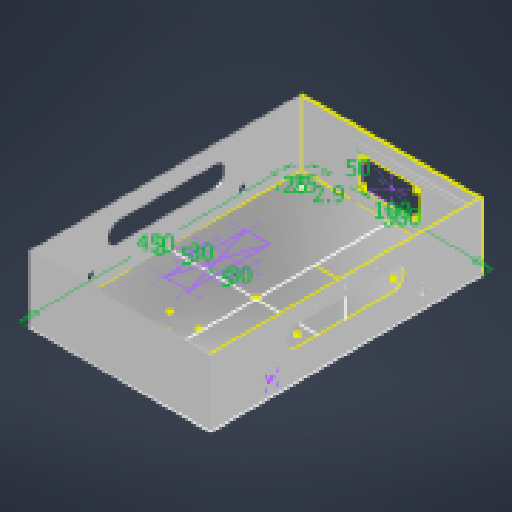
# Autodesk Inventor part: AMR_Base_Box_V2
Saved by Autodesk Inventor 2026.2 (Build 302298010, 298A)
## iProperties
Created: 2026-03-25
Part Number: AMR_Base_Box_V2
Material: Aluminum 6061
Document SubType Name: Modeling
Designer: Srishanth Dhondy
Density: 2.7 g/cm^3
Appearance: Aluminum - Flat
Mass: 2297.89 g
Surface Area: 5654.69 cm^2
Volume: 851.072 cm^3
Author: Srishanth Dhondy
Autodesk Inventor part; units mm, degrees
ref_plane "YZ Plane" through (0, 0, 0) normal (1, 0, 0) x (0, 1, 0)
ref_plane "XZ Plane" through (0, 0, 0) normal (0, 1, 0) x (-1, 0, 0)
ref_plane "XY Plane" through (0, 0, 0) normal (0, 0, 1) x (1, 0, 0)
sketch "Sketch1" plane through (0, 0, 0) normal (0, 1, 0) x (-1, 0, 0)
  line L0 (-150, 225) -> (150, 225)
  line L1 (150, 225) -> (150, -225)
  line L2 (150, -225) -> (-150, -225)
  line L3 (-150, -225) -> (-150, 225)
  line L4 (-150, 225) -> (150, -225) construction
  line L5 (150, 225) -> (-150, -225) construction
  line L6 (147, -222) -> (147, 222)
  line L7 (147, 222) -> (-147, 222)
  line L8 (-147, 222) -> (-147, -222)
  line L9 (-147, -222) -> (147, -222)
  point P0 (0, 0)
  dimension "Base_Width" = 300
  dimension "Base_Length" = 450
  dimension "Base_Wall_Thickness" = 3
  constraints: 20 end point, 4 parallel, 2 midpoint, 2 perpendicular, 1 horizontal, 3 other
  measures "Base_Width" distance of L1.end L2.end
  measures "Base_Length" distance of L0.end L1.end
  measures "Base_Wall_Thickness" distance between parallel lines of L1 L6
extrude "Extrusion1" add sketch "Sketch1" along normal blind 3 contours L0 L1 L2 L3 | L9 L8 L7 L6
extrude "Extrusion2" add sketch "Sketch1" along normal blind 110
sketch "Sketch2" plane through (150, 0, 225) normal (1, 0, 0) x (0, 0, -1)
  line L0 (0, 0) -> (450, 0) projected
  line L1 (450, 0) -> (450, 110) projected
  line L2 (0, 110) -> (450, 110) projected
  line L3 (0, 0) -> (0, 110) projected
  line L4 (0, 25) -> (450, 25)
  line L5 (100, 25) -> (114, 25) construction
  line L6 (225, 110) -> (225, 0) construction
  circle A0 centre (100, 25) radius 19.5
  circle A1 centre (100, 25) radius 6
  circle A2 centre (100, 25) radius 7.75
  circle A3 centre (84.5, 25) radius 1.75
  circle A4 centre (100, 40.5) radius 1.75
  circle A5 centre (100, 9.5) radius 1.75
  circle A6 centre (115.5, 25) radius 1.75
  line L7 (350, 25) -> (336, 25) construction
  circle A7 centre (350, 25) radius 19.5
  circle A8 centre (350, 25) radius 6
  circle A9 centre (350, 25) radius 7.75
  circle A10 centre (365.5, 25) radius 1.75
  circle A11 centre (350, 40.5) radius 1.75
  circle A12 centre (350, 9.5) radius 1.75
  circle A13 centre (334.5, 25) radius 1.75
  point P0 (119.5, 25)
  point P1 (80.5, 25)
  point P2 (100, 5.5)
  point P3 (100, 44.5)
  point P4 (330.5, 25)
  point P5 (369.5, 25)
  point P6 (350, 5.5)
  point P7 (350, 44.5)
  dimension "d138" = 39
  dimension "d139" = 12
  dimension "d140" = 15.5
  dimension "d141" = 3.5
  dimension "d143" = 3.5
  dimension "d144" = 3.5
  dimension "d145" = 3.5
  constraints: 22 coincident, 22 symmetric about line, 14 centre point, 8 end point, 8 point on circle, 7 point on line, 2 perpendicular, 1 horizontal, 1 midpoint, 7 other
  measures "d138" diameter of A0
  measures "d139" diameter of A1
  measures "d140" diameter of A2
  measures "d141" diameter of A3
  measures "d143" diameter of A4
  measures "d144" diameter of A5
  measures "d145" diameter of A6
sketch "Sketch3" plane through (0, 3, 0) normal (0, 1, 0) x (1, 0, 0)
  line L0 (-147, 222) -> (-147, -222) projected
  line L1 (-147, -222) -> (147, -222) projected
  line L2 (147, -222) -> (147, 222) projected
  line L3 (147, 222) -> (-147, 222) projected
  point P0 (0, 0)
sketch "Sketch7" plane through (150, 0, 225) normal (1, 0, 0) x (0, 0, -1)
  line L0 (145, 65.000074) -> (305, 65.000074) construction
  line L1 (145, 47.500074) -> (305, 47.500074)
  line L2 (305, 82.500074) -> (145, 82.500074)
  arc A0 (145, 82.500074) -> (145, 47.500074) centre (145, 65.000074) ccw
  arc A1 (305, 47.500074) -> (305, 82.500074) centre (305, 65.000074) ccw
  point P0 (225, 0)
  point P1 (225, 65.000074)
  dimension "Handle_Slot_Length" = 80
  dimension "Handle_Cutout_Height" = 35
  constraints: 8 end point, 4 point on circle, 4 tangent, 2 centre point, 1 horizontal, 1 midpoint, 1 parallel
  measures "Handle_Slot_Length" distance of point (225, 65) L0.end
  measures "Handle_Cutout_Height" diameter of A1
extrude "Extrusion3" cut sketch "Sketch7" against normal through all
sketch "Sketch9" plane through (150, 0, -225) normal (0, 0, -1) x (-1, 0, 0)
  line L0 (0, 0) -> (300, 0) projected
  line L1 (300, 0) -> (300, 110) projected
  line L2 (0, 110) -> (300, 110) projected
  line L3 (0, 0) -> (0, 110) projected
  line L4 (100, 75) -> (200, 75)
  line L5 (200, 75) -> (200, 25)
  line L6 (200, 25) -> (100, 25)
  line L7 (100, 25) -> (100, 75)
  line L8 (100, 75) -> (200, 25) construction
  line L9 (200, 75) -> (100, 25) construction
  point P0 (150, 0)
  point P1 (150, 50)
  point P2 (150, 50)
  dimension "Rear_Port_Width" = 100
  dimension "Rear_Port_Height" = 50
  constraints: 12 end point, 2 midpoint, 2 parallel, 1 coincident, 1 horizontal, 1 perpendicular
  measures "Rear_Port_Width" distance of L5.end L6.end
  measures "Rear_Port_Height" distance of L4.end L5.end
sketch "Sketch10" plane through (150, 0, -225) normal (0, 0, -1) x (-1, 0, 0)
  line L0 (100.000061, 70.00003) -> (100.000061, 30.000011)
  line L1 (105.000061, 25.000011) -> (195.003813, 25.000011)
  line L2 (200.003813, 30.000011) -> (200.003813, 70.00003)
  line L3 (195.003813, 75.00003) -> (105.000061, 75.00003)
  arc A0 (105.000061, 75.00003) -> (100.000061, 70.00003) centre (105.000061, 70.00003) ccw
  arc A1 (100.000061, 30.000011) -> (105.000061, 25.000011) centre (105.000061, 30.000011) ccw
  arc A2 (195.003813, 25.000011) -> (200.003813, 30.000011) centre (195.003813, 30.000011) ccw
  arc A3 (200.003813, 70.00003) -> (195.003813, 75.00003) centre (195.003813, 70.00003) ccw
  point P0 (150, 0)
  point P1 (200.003813, 75.00003)
  point P2 (100.003813, 75.00003)
  dimension "d48" = 100
  dimension "Rear_Port_Fillet" = 5
  constraints: 8 end point, 8 point on circle, 8 tangent, 4 centre point, 3 equal radius, 3 perpendicular, 3 point on line, 1 vertical
  measures "d48" distance of point (200.004, 75) point (100.004, 75)
  measures "Rear_Port_Fillet" radius of A0
extrude "Extrusion4" cut sketch "Sketch10" against normal blind 3
sketch "Sketch11" plane through (147, 3, 222) normal (-1, 0, 0) x (0, 0, 1)
  line L0 (-302, 79.500074) -> (-142, 79.500074)
  arc A0 (-142, 44.500074) -> (-142, 79.500074) centre (-142, 62.000074) ccw
  line L1 (-142, 44.500074) -> (-302, 44.500074)
  arc A1 (-302, 79.500074) -> (-302, 44.500074) centre (-302, 62.000074) ccw
  circle A2 centre (-106.899495, 31.899495) radius 1.75
  circle A3 centre (-87.100505, 12.100505) radius 1.75
  circle A4 centre (-106.899495, 12.100505) radius 1.75
  circle A5 centre (-87.100505, 31.899495) radius 1.75
  circle A6 centre (-97, 22) radius 6
  line L2 (0, 0) -> (-444, 0)
  line L3 (0, 0) -> (0, 107)
  line L4 (-444, 107) -> (0, 107)
  line L5 (-444, 0) -> (-444, 107)
  line L6 (0, 107) -> (-444, 107)
  line L7 (-222, 107) -> (-222, -3)
  line L8 (-222, -3) -> (-222, 107)
  constraints: 4 end point, 2 perpendicular, 1 midpoint
sketch "Sketch13" plane through (-147, 3, -222) normal (0, 0, 1) x (1, 0, 0)
  line L0 (191.999939, 22.000011) -> (101.996187, 22.000011)
  arc A0 (96.996187, 27.000011) -> (101.996187, 22.000011) centre (101.996187, 27.000011) ccw
  line L1 (96.996187, 27.000011) -> (96.996187, 67.00003)
  arc A1 (101.996187, 72.00003) -> (96.996187, 67.00003) centre (101.996187, 67.00003) ccw
  line L2 (101.996187, 72.00003) -> (191.999939, 72.00003)
  arc A2 (196.999939, 67.00003) -> (191.999939, 72.00003) centre (191.999939, 67.00003) ccw
  line L3 (196.999939, 67.00003) -> (196.999939, 27.000011)
  arc A3 (191.999939, 22.000011) -> (196.999939, 27.000011) centre (191.999939, 27.000011) ccw
  line L4 (294, 0) -> (0, 0)
  line L5 (294, 0) -> (294, 107)
  line L6 (0, 107) -> (294, 107)
  line L7 (0, 0) -> (0, 107)
  point P0 (147, -3)
sketch "Sketch14" plane through (-147, 3, -222) normal (0, 0, 1) x (1, 0, 0)
  line L0 (294, 0) -> (0, 0)
  line L1 (294, 0) -> (294, 107)
  line L2 (0, 0) -> (0, 107)
  line L3 (297, 107) -> (-3, 107)
  line L4 (147, 107) -> (147, 0)
  line L5 (101.996187, 13.5) -> (293.998542, 13.5)
  line L6 (293.998542, 13.5) -> (293.998542, 3.5)
  line L7 (293.998542, 3.5) -> (101.996187, 3.5)
  line L8 (101.996187, 3.5) -> (101.996187, 13.5)
  line L9 (0, 53.5) -> (294, 53.5)
  line L10 (101.996187, 90.5) -> (293.996187, 90.5)
  line L11 (293.996187, 90.5) -> (293.996187, 80.5)
  line L12 (293.996187, 80.5) -> (101.996187, 80.5)
  line L13 (101.996187, 80.5) -> (101.996187, 90.5)
  point P0 (101.996187, 22.000011)
  point P1 (147, -3)
  point P2 (101.996187, 22.000011)
  point P3 (0.001458, 3.5)
  point P4 (0.001458, 3.5)
  point P5 (192.003813, 13.5)
  point P6 (0.003813, 80.5)
  point P7 (0.003813, 80.5)
  point P8 (192.003813, 90.5)
  dimension "d52" = 192
  dimension "d53" = 10
  constraints: 20 end point, 5 coincident, 4 midpoint, 4 parallel, 4 symmetric about line, 2 horizontal, 2 perpendicular, 1 point on line
  measures "d52" distance of L11.end L12.end
  measures "d53" distance of L12.end L10.start
sketch "Sketch14 outline for Extrusion5" plane through (-147, 3, -222) normal (0, 0, 1) x (1, 0, 0)
  line L0 (293.998542, 3.5) -> (293.998542, 13.5)
  line L1 (101.996187, 3.5) -> (293.998542, 3.5)
  line L2 (101.996187, 13.5) -> (101.996187, 3.5)
  line L3 (293.998542, 13.5) -> (101.996187, 13.5)
  line L4 (293.996187, 80.5) -> (293.996187, 90.5)
  line L5 (101.996187, 80.5) -> (293.996187, 80.5)
  line L6 (101.996187, 90.5) -> (101.996187, 80.5)
  line L7 (293.996187, 90.5) -> (101.996187, 90.5)
extrude "Extrusion5" add sketch "Sketch14 outline for Extrusion5" along normal blind 3.5
sketch "Sketch15" plane through (-147, 3, -218.5) normal (0, 0, 1) x (1, 0, 0)
  line L0 (101.996187, 90.5) -> (101.996187, 80.5)
  line L1 (101.996187, 80.5) -> (293.996187, 80.5)
  line L2 (293.996187, 80.5) -> (293.996187, 90.5)
  line L3 (101.996187, 85.5) -> (293.996187, 85.5)
  line L4 (293.996187, 85.5) -> (293.996187, 80.5)
  line L5 (293.996187, 80.5) -> (101.996187, 80.5)
  line L6 (101.996187, 80.5) -> (101.996187, 85.5)
  line L7 (293.998542, 13.5) -> (101.996187, 13.5)
  line L8 (293.998542, 3.5) -> (293.998542, 13.5)
  line L9 (101.996187, 13.5) -> (293.998542, 13.5)
  line L10 (293.998542, 13.5) -> (293.998542, 8.5)
  line L11 (293.998542, 8.5) -> (101.996187, 8.5)
  line L12 (101.996187, 8.5) -> (101.996187, 13.5)
  point P0 (147, -3)
  constraints: 16 end point, 4 parallel, 2 horizontal, 2 midpoint, 2 perpendicular
extrude "Extrusion6" add sketch "Sketch15" along normal blind 2
sketch "Sketch17" plane through (0, 3, 0) normal (0, 1, 0) x (1, 0, 0)
  line L0 (-147, 222) -> (-147, -222) projected
  line L1 (-147, -222) -> (147, -222) projected
  line L2 (147, -222) -> (147, 222) projected
  line L3 (147, 222) -> (-147, 222) projected
  circle A0 centre (-120.55, 195.55) radius 1.45
  line L4 (-147, 0) -> (147, 0)
  line L5 (0, -222) -> (0, 222)
  circle A1 centre (-120.55, -195.55) radius 1.45
  line L6 (0, 222) -> (0, -222)
  circle A2 centre (-120.55, -195.55) radius 1.45
  circle A3 centre (120.55, 195.55) radius 1.45
  circle A4 centre (120.55, -195.55) radius 1.45
  line L7 (0, 222) -> (0, -222)
  point P0 (0, 0)
  dimension "d58" = 2.9
  dimension "d59" = 25
  dimension "d60" = 25
  constraints: 8 end point, 6 symmetric about line, 5 centre point, 4 midpoint, 1 perpendicular, 4 other
  measures "d58" diameter of A0
  measures "d59" distance edge to line of A0 L3
  measures "d60" distance edge to line of A0 L0
extrude "Extrusion7" cut sketch "Sketch17" against normal blind 110 contours A0
extrude "Extrusion8" cut sketch "Sketch17" against normal blind 110 contours A1
extrude "Extrusion9" cut sketch "Sketch17" against normal blind 110 contours A4
extrude "Extrusion10" cut sketch "Sketch17" against normal blind 110 contours A3
sketch "Sketch18" plane through (-147, 3, -222) normal (1, 0, 0) x (0, 0, -1)
  line L0 (-142, 79.500074) -> (-285.5, 79.500074)
  line L1 (-285.5, 79.500074) -> (-285.5, 101.1)
  line L2 (-158.5, 79.503299) -> (-285.5, 79.503299)
  line L3 (-285.5, 79.503299) -> (-285.5, 102.503299)
  line L4 (-285.5, 102.503299) -> (-158.5, 102.503299)
  line L5 (-158.5, 102.503299) -> (-158.5, 79.503299)
  line L6 (-158.5, 79.503299) -> (-285.5, 102.503299) construction
  line L7 (-285.5, 79.503299) -> (-158.5, 102.503299) construction
  circle A0 centre (-272.8, 92.853299) radius 2.25
  circle A1 centre (-171.2, 92.978299) radius 2.25
  point P0 (-222, -3)
  point P1 (-302, 101.1)
  point P2 (-302, 101.1)
  point P3 (-302, 101.1)
  point P4 (-302, 101.1)
  point P5 (-142, 101.1)
  point P6 (-142, 101.1)
  point P7 (-142, 101.1)
  point P8 (-158.5, 101.1)
  point P9 (-222, 93.25)
  point P10 (-222, 91.003299)
  dimension "d70" = 127
  dimension "d71" = 23
  dimension "d73" = 4.5
  dimension "d74" = 11.1
  dimension "d75" = 12.7
  dimension "d76" = 4.5
  dimension "d77" = 13.475
  dimension "d78" = 12.7
  constraints: 16 end point, 5 coincident, 2 centre point, 2 midpoint, 2 parallel, 1 horizontal, 1 perpendicular
  measures "d70" distance of L3.end L4.end
  measures "d71" distance of L2.end L3.end
  measures "d73" diameter of A0
  measures "d74" distance edge to line of A0 L2
  measures "d75" distance from line of L3 A0.centre
  measures "d76" diameter of A1
  measures "d77" distance from line of L2 A1.centre
  measures "d78" distance from line of L5 A1.centre
extrude "Extrusion11" cut sketch "Sketch18" along normal through all both and the other way through all contours A0 | A1
sketch "Sketch19" plane through (-147, 3, -222) normal (1, 0, 0) x (0, 0, -1)
  circle A0 centre (-222, 92.978299) radius 2.25
  point P0 (-222, -3)
  dimension "d81" = 4.5
  constraints: 1 centre point, 1 coincident
  measures "d81" diameter of A0
extrude "Extrusion12" cut sketch "Sketch19" along normal through all both and the other way through all
sketch "Sketch22" plane through (147, 3, 222) normal (-1, 0, 0) x (0, 0, 1)
  line L0 (-444, 0) -> (-444, 107) projected
  line L1 (-444, 80.5) -> (-440.5, 80.5)
  line L2 (-440.5, 80.5) -> (-440.5, 13.5)
  line L3 (-440.5, 13.5) -> (-444, 13.5)
  line L4 (-444, 13.5) -> (-444, 80.5)
  point P0 (-222, -3)
  dimension "d84" = 3.5
  constraints: 8 end point, 2 parallel, 1 horizontal, 1 perpendicular
  measures "d84" distance of L2.end L3.end
extrude "Extrusion13" add sketch "Sketch22" along normal blind 10
sketch "Sketch23" plane through (-147, 110, -222) normal (0, 0, 1) x (1, 0, 0)
  line L0 (101.996187, -26.5) -> (101.996187, -16.5)
  line L1 (101.996187, -26.5) -> (293.996187, -26.5)
  line L2 (101.996187, -26.5) -> (95.696187, -26.5)
  line L3 (95.696187, -26.5) -> (95.696187, -16.5)
  line L4 (95.696187, -16.5) -> (101.996187, -16.5)
  line L5 (101.996187, -16.5) -> (101.996187, -26.5)
  line L6 (101.996187, -21.5) -> (293.996187, -21.5)
  line L7 (101.996187, -21.5) -> (105.795872, -23.663742)
  line L8 (101.996187, -21.5) -> (95.696187, -21.5)
  line L9 (95.696187, -21.5) -> (101.996187, -21.5)
  point P0 (147, -110)
  dimension "d87" = 6.3
  dimension "d88" = 10
  dimension "d89" = 6.3
  constraints: 14 end point, 2 parallel, 1 horizontal, 1 midpoint, 1 perpendicular
  measures "d87" distance of L3.end L4.end
  measures "d88" distance of L2.end L3.end
  measures "d89" distance of L6.start L8.end
extrude "Extrusion14" add sketch "Sketch23" along normal blind 5.5 contours L2 L3 L8 L0
extrude "Extrusion15" add sketch "Sketch23" along normal blind 3.5
sketch "Sketch24" plane through (-147, 110, -222) normal (0, 0, 1) x (1, 0, 0)
  line L0 (101.996187, -103.5) -> (101.996187, -93.5)
  line L1 (101.996187, -103.5) -> (95.696187, -103.5)
  line L2 (95.696187, -103.5) -> (95.696187, -93.5)
  line L3 (95.696187, -93.5) -> (101.996187, -93.5)
  line L4 (101.996187, -93.5) -> (101.996187, -103.5)
  line L5 (101.996187, -98.5) -> (105.945782, -102.881271)
  line L6 (101.996187, -98.5) -> (95.696, -98.5)
  point P0 (147, -110)
  point P1 (95.696187, -98.5)
  dimension "d94" = 6.3
  constraints: 12 end point, 2 parallel, 2 perpendicular, 1 horizontal, 1 midpoint
  measures "d94" distance of L2.end L3.end
extrude "Extrusion16" add sketch "Sketch24" along normal blind 5.5 contours L6 L2 L3 L0
extrude "Extrusion17" add sketch "Sketch24" along normal blind 3.5 contours L1 L2 L6 L0
sketch "Sketch25" plane through (-147, 110, -222) normal (0, 0, 1) x (1, 0, 0)
  line L0 (95.696187, -103.5) -> (95.696187, -93.5)
  line L1 (95.696187, -93.5) -> (284, -93.5)
  line L2 (284, -26.5) -> (95.696187, -26.5)
  line L3 (95.696187, -26.5) -> (95.696187, -16.5)
  line L4 (95.696187, -16.5) -> (293.996187, -16.5)
  line L5 (293.998542, -103.5) -> (95.696187, -103.5)
  line L6 (95.696187, -103.5) -> (85.696, -103.5)
  line L7 (85.696, -103.5) -> (85.696, -16.5)
  line L8 (85.696, -16.5) -> (95.696187, -16.5)
  line L9 (95.696187, -16.5) -> (95.696187, -103.5)
  point P0 (147, -110)
  point P1 (85.696, -26.5)
  point P2 (85.696, -93.5)
  point P3 (85.696, -100.25)
  constraints: 8 end point, 4 point on line, 2 parallel, 1 horizontal, 1 perpendicular
extrude "Extrusion18" add sketch "Sketch25" along normal blind 5.5
sketch "Sketch26" plane through (0, 3, 0) normal (0, 1, 0) x (1, 0, 0)
  line L0 (-1.867084, -74) -> (-51.867084, -74)
  line L1 (-54.867084, -77) -> (-54.867084, -150)
  line L2 (-51.867084, -153) -> (-1.867084, -153)
  line L3 (1.132916, -150) -> (1.132916, -77)
  arc A0 (-54.867084, -150) -> (-51.867084, -153) centre (-51.867084, -150) ccw
  arc A1 (-1.867084, -153) -> (1.132916, -150) centre (-1.867084, -150) ccw
  arc A2 (1.132916, -77) -> (-1.867084, -74) centre (-1.867084, -77) ccw
  arc A3 (-51.867084, -74) -> (-54.867084, -77) centre (-51.867084, -77) ccw
  line L4 (-26.867084, -74) -> (-26.867084, -153)
  line L5 (-54.867084, -113.5) -> (1.132916, -113.5)
  circle A4 centre (-51.367, -149.5) radius 1.35
  circle A5 centre (-2.367168, -149.5) radius 1.35
  circle A6 centre (-51.367, -77.5) radius 1.35 construction
  circle A7 centre (-2.367168, -77.5) radius 1.35
  circle A8 centre (-2.367168, -77.5) radius 1.35
  circle A9 centre (-51.367, -149.5) radius 1.35
  circle A10 centre (-2.367168, -149.5) radius 1.35
  circle A11 centre (-51.367, -77.5) radius 1.35
  line L6 (-51.367, -77.5) -> (-51.367, -149.5)
  circle A12 centre (-51.367, -91.5) radius 1.35
  circle A13 centre (-2.367168, -91.5) radius 1.35
  point P0 (0, 0)
  point P1 (-64, -151.953345)
  point P2 (-14, -151.953345)
  point P3 (-54.867084, -153)
  point P4 (-54.867084, -74)
  point P5 (-60.5, -150)
  point P6 (-61, -149.5)
  point P7 (-51.367, -150)
  point P8 (-51.867084, -149.5)
  point P9 (-51.367, -77.564433)
  dimension "d101" = 79
  dimension "d102" = 3
  dimension "d103" = 3
  dimension "d104" = 3
  dimension "d105" = 3
  dimension "d109" = 50
  dimension "d111" = 2.7
  dimension "d114" = 2.7
  constraints: 14 centre point, 14 end point, 8 point on circle, 8 tangent, 7 coincident, 6 point on line, 4 concentric, 4 midpoint, 4 symmetric about line, 2 parallel, 1 horizontal, 1 perpendicular, 4 other
  measures "d101" distance of point (-54.867, -153) point (-54.867, -74)
  measures "d102" radius of A0
  measures "d103" radius of A1
  measures "d104" radius of A2
  measures "d105" radius of A3
  measures "d109" distance of L2.end L2.start
  measures "d111" diameter of A4
  measures "d114" diameter of A12
extrude "Extrusion21" cut sketch "Sketch26" against normal through all contours A4 | A5 | A12 L6 | L6 A12 | A13
sketch "Sketch28" plane through (0, 3, 0) normal (0, 1, 0) x (1, 0, 0)
  line L0 (0, 97) -> (53, 97)
  line L1 (53, 97) -> (53, 0)
  line L2 (53, 0) -> (0, 0)
  line L3 (0, 0) -> (0, 97)
  constraints: 8 end point, 2 parallel, 1 horizontal, 1 perpendicular
sketch "Sketch29" plane through (0, 3, 0) normal (0, 1, 0) x (1, 0, 0)
  line L0 (-147, -222) -> (147, -222)
  line L1 (147, -222) -> (147, 222)
  line L2 (147, 222) -> (-147, 222)
  circle A0 centre (-120.55, 195.55) radius 1.45
  line L3 (-126.3, 201.3) -> (-114.8, 201.3)
  line L4 (-114.8, 201.3) -> (-114.8, 189.8)
  line L5 (-114.8, 189.8) -> (-126.3, 189.8)
  line L6 (-126.3, 189.8) -> (-126.3, 201.3)
  line L7 (-120.55, 195.55) -> (-126.489697, 201.489697)
  line L8 (-120.55, 195.55) -> (-114.610303, 201.489697)
  line L9 (-120.55, 195.55) -> (-126.489697, 189.610303)
  line L10 (-120.55, 195.55) -> (-114.610303, 189.610303)
  line L11 (0, 222) -> (0, -222)
  line L12 (147, 0) -> (-150, 0)
  line L13 (-150, 225) -> (-150, -225)
  line L14 (-126.489697, 201.489697) -> (-114.610303, 201.489697)
  line L15 (-114.610303, 201.489697) -> (-114.610303, 189.610303)
  line L16 (-114.610303, 189.610303) -> (-126.489697, 189.610303)
  line L17 (-126.489697, 189.610303) -> (-126.489697, 201.489697)
  line L18 (114.610303, 201.489697) -> (126.489697, 201.489697)
  line L19 (126.489697, 201.489697) -> (126.489697, 189.610303)
  line L20 (126.489697, 189.610303) -> (114.610303, 189.610303)
  line L21 (114.610303, 189.610303) -> (114.610303, 201.489697)
  line L22 (-126.489697, -189.610303) -> (-114.610303, -189.610303)
  line L23 (-114.610303, -189.610303) -> (-114.610303, -201.489697)
  line L24 (-114.610303, -201.489697) -> (-126.489697, -201.489697)
  line L25 (-126.489697, -201.489697) -> (-126.489697, -189.610303)
  line L26 (114.610303, -189.610303) -> (126.489697, -189.610303)
  line L27 (126.489697, -189.610303) -> (126.489697, -201.489697)
  line L28 (126.489697, -201.489697) -> (114.610303, -201.489697)
  line L29 (114.610303, -201.489697) -> (114.610303, -189.610303)
  point P0 (0, 0)
  point P1 (126.489697, 201.489697)
  point P2 (114.610303, 189.610303)
  point P3 (-126.489697, -201.489697)
  point P4 (-114.610303, -189.610303)
  point P5 (114.610303, -201.489697)
  point P6 (126.489697, -189.610303)
  dimension "d121" = 5.75
  dimension "d122" = 5.75
  dimension "d123" = 5.75
  dimension "d124" = 5.75
  dimension "d125" = 5.75
  dimension "d126" = 5.75
  dimension "d127" = 8.4
  dimension "d128" = 8.4
  dimension "d129" = 8.4
  dimension "d130" = 8.4
  constraints: 52 end point, 13 coincident, 12 symmetric about line, 10 parallel, 6 perpendicular, 5 horizontal, 4 midpoint
  measures "d121" horizontal distance of L7.start point (-126.3, 201.3)
  measures "d122" horizontal distance of L7.start point (-126.3, 189.8)
  measures "d123" horizontal distance of L7.start point (-126.3, 201.3)
  measures "d124" horizontal distance of L7.start point (-126.3, 189.8)
  measures "d125" horizontal distance of L7.start point (-114.8, 201.3)
  measures "d126" horizontal distance of L7.start point (-114.8, 189.8)
  measures "d127" distance of L7.start L7.end
  measures "d128" distance of L7.start L8.end
  measures "d129" distance of L7.start L9.end
  measures "d130" distance of L7.start L10.end
sketch "Sketch30" plane through (0, 3, 0) normal (0, 1, 0) x (1, 0, 0)
  circle A0 centre (-51.367, -91.5) radius 1.35
  circle A1 centre (-2.367168, -149.5) radius 1.35
  circle A2 centre (-2.367168, -91.5) radius 1.35
  circle A3 centre (-51.367, -149.5) radius 1.35
  circle A4 centre (120.55, 195.55) radius 1.45
  circle A5 centre (120.55, -195.55) radius 1.45
  circle A6 centre (-120.55, -195.55) radius 1.45
  circle A7 centre (-120.55, 195.55) radius 1.45
  line L0 (-147, 222) -> (-147, -222)
  line L1 (-147, -222) -> (147, -222)
  line L2 (147, -222) -> (147, 222)
  line L3 (147, 222) -> (-147, 222)
  point P0 (0, 0)
split_face "Split1"
split_face "Split2"
split_face "Split3"
split_face "Split4"
extrude "Extrusion25" cut sketch "Sketch2" against normal through all contours A3 L4 | L4 A3 | A10 L4 | L4 A10 | A6 L4 | L4 A6 | A13 L4 | L4 A13 | A1 L4 | L4 A1 | A8 L4 | L4 A8 | A4 | A5 | A11 | A12
split_face "Split5"
sketch "Sketch31" plane through (-147, 3, 222) normal (0, 1, 0) x (1, 0, 0)
  line L0 (32.389697, 20.510303) -> (32.389697, 32.389697)
  line L1 (20.510303, 20.510303) -> (32.389697, 20.510303)
  line L2 (20.510303, 32.389697) -> (20.510303, 20.510303)
  line L3 (32.389697, 32.389697) -> (20.510303, 32.389697)
  line L4 (273.489697, 411.610303) -> (273.489697, 423.489697)
  line L5 (261.610303, 411.610303) -> (273.489697, 411.610303)
  line L6 (261.610303, 423.489697) -> (261.610303, 411.610303)
  line L7 (273.489697, 423.489697) -> (261.610303, 423.489697)
  line L8 (0, 444) -> (0, 0)
  line L9 (0, 0) -> (294, 0)
  line L10 (294, 0) -> (294, 444)
  line L11 (294, 444) -> (0, 444)
  circle A0 centre (95.633, 72.5) radius 1.35
  circle A1 centre (144.632832, 130.5) radius 1.35
  circle A2 centre (144.632832, 72.5) radius 1.35
  circle A3 centre (95.633, 130.5) radius 1.35
  line L12 (20.510303, 411.610303) -> (32.389697, 411.610303)
  line L13 (20.510303, 423.489697) -> (20.510303, 411.610303)
  line L14 (32.389697, 423.489697) -> (20.510303, 423.489697)
  line L15 (32.389697, 411.610303) -> (32.389697, 423.489697)
  line L16 (273.489697, 20.510303) -> (273.489697, 32.389697)
  line L17 (261.610303, 20.510303) -> (273.489697, 20.510303)
  line L18 (261.610303, 32.389697) -> (261.610303, 20.510303)
  line L19 (273.489697, 32.389697) -> (261.610303, 32.389697)
  line L20 (200, 319) -> (147, 319)
  line L21 (200, 222) -> (200, 319)
  line L22 (147, 222) -> (200, 222)
  line L23 (147, 319) -> (147, 222)
sketch "Sketch32" plane through (-147, 3, 222) normal (0, 1, 0) x (1, 0, 0)
  line L0 (32.389697, 20.510303) -> (32.389697, 32.389697)
  line L1 (20.510303, 20.510303) -> (32.389697, 20.510303)
  line L2 (20.510303, 32.389697) -> (20.510303, 20.510303)
  line L3 (32.389697, 32.389697) -> (20.510303, 32.389697)
  line L4 (273.489697, 411.610303) -> (273.489697, 423.489697)
  line L5 (261.610303, 411.610303) -> (273.489697, 411.610303)
  line L6 (261.610303, 423.489697) -> (261.610303, 411.610303)
  line L7 (273.489697, 423.489697) -> (261.610303, 423.489697)
  line L8 (0, 444) -> (0, 0)
  line L9 (0, 0) -> (294, 0)
  line L10 (294, 0) -> (294, 444)
  line L11 (294, 444) -> (0, 444)
  circle A0 centre (95.633, 72.5) radius 1.35
  circle A1 centre (144.632832, 130.5) radius 1.35
  circle A2 centre (144.632832, 72.5) radius 1.35
  circle A3 centre (95.633, 130.5) radius 1.35
  line L12 (20.510303, 411.610303) -> (32.389697, 411.610303)
  line L13 (20.510303, 423.489697) -> (20.510303, 411.610303)
  line L14 (32.389697, 423.489697) -> (20.510303, 423.489697)
  line L15 (32.389697, 411.610303) -> (32.389697, 423.489697)
  line L16 (273.489697, 20.510303) -> (273.489697, 32.389697)
  line L17 (261.610303, 20.510303) -> (273.489697, 20.510303)
  line L18 (261.610303, 32.389697) -> (261.610303, 20.510303)
  line L19 (273.489697, 32.389697) -> (261.610303, 32.389697)
  line L20 (200, 319) -> (147, 319)
  line L21 (200, 222) -> (200, 319)
  line L22 (147, 222) -> (200, 222)
  line L23 (147, 319) -> (147, 222)
  line L24 (39.618491, 312.252) -> (79.6, 312.252)
  line L25 (79.6, 312.252) -> (79.6, 178.252222)
  line L26 (79.6, 178.252222) -> (39.618491, 178.252222)
  line L27 (39.618491, 178.252222) -> (39.618491, 312.252)
  constraints: 8 end point, 2 parallel, 1 horizontal, 1 perpendicular
sketch "Sketch33" plane through (-147, 3, 222) normal (0, 1, 0) x (1, 0, 0)
  line L0 (32.389697, 20.510303) -> (32.389697, 32.389697)
  line L1 (20.510303, 20.510303) -> (32.389697, 20.510303)
  line L2 (20.510303, 32.389697) -> (20.510303, 20.510303)
  line L3 (32.389697, 32.389697) -> (20.510303, 32.389697)
  line L4 (273.489697, 411.610303) -> (273.489697, 423.489697)
  line L5 (261.610303, 411.610303) -> (273.489697, 411.610303)
  line L6 (261.610303, 423.489697) -> (261.610303, 411.610303)
  line L7 (273.489697, 423.489697) -> (261.610303, 423.489697)
  line L8 (0, 444) -> (0, 0)
  line L9 (0, 0) -> (294, 0)
  line L10 (294, 0) -> (294, 444)
  line L11 (294, 444) -> (0, 444)
  circle A0 centre (95.633, 72.5) radius 1.35
  circle A1 centre (144.632832, 130.5) radius 1.35
  circle A2 centre (144.632832, 72.5) radius 1.35
  circle A3 centre (95.633, 130.5) radius 1.35
  line L12 (20.510303, 411.610303) -> (32.389697, 411.610303)
  line L13 (20.510303, 423.489697) -> (20.510303, 411.610303)
  line L14 (32.389697, 423.489697) -> (20.510303, 423.489697)
  line L15 (32.389697, 411.610303) -> (32.389697, 423.489697)
  line L16 (273.489697, 20.510303) -> (273.489697, 32.389697)
  line L17 (261.610303, 20.510303) -> (273.489697, 20.510303)
  line L18 (261.610303, 32.389697) -> (261.610303, 20.510303)
  line L19 (273.489697, 32.389697) -> (261.610303, 32.389697)
  line L20 (200, 319) -> (147, 319)
  line L21 (200, 222) -> (200, 319)
  line L22 (147, 222) -> (200, 222)
  line L23 (147, 319) -> (147, 222)
  line L24 (39.618489, 312.251998) -> (79.6, 178.252204)
  line L25 (79.6, 312.251998) -> (39.618489, 178.252204)
  point P0 (59.609244, 245.252101)
  constraints: 4 end point, 1 midpoint
sketch "Sketch34" plane through (-147, 3, 222) normal (0, 1, 0) x (1, 0, 0)
  circle A0 centre (95.633, 72.5) radius 1.35
  circle A1 centre (144.632832, 130.5) radius 1.35
  circle A2 centre (144.632832, 72.5) radius 1.35
  circle A3 centre (95.633, 130.5) radius 1.35
  line L0 (95.633, 130.5) -> (144.632832, 72.5)
  line L1 (144.632832, 130.5) -> (95.633, 72.5)
  circle A4 centre (120.132916, 101.5) radius 2.5
  dimension "d148" = 5
  constraints: 4 end point, 1 centre point, 1 coincident, 1 midpoint
  measures "d148" diameter of A4
extrude "Extrusion26" add sketch "Sketch34" along normal blind 5 contours A4 L1 L0 | L0 L1 A4 | L1 A4 L0 | L0 A4 L1
sketch "Sketch35" plane through (-147, 3, 222) normal (0, 1, 0) x (1, 0, 0)
  circle A0 centre (120.132916, 101.5) radius 2.5
  line L0 (32.389697, 20.510303) -> (32.389697, 32.389697)
  line L1 (20.510303, 20.510303) -> (32.389697, 20.510303)
  line L2 (20.510303, 32.389697) -> (20.510303, 20.510303)
  line L3 (32.389697, 32.389697) -> (20.510303, 32.389697)
  line L4 (273.489697, 411.610303) -> (273.489697, 423.489697)
  line L5 (261.610303, 411.610303) -> (273.489697, 411.610303)
  line L6 (261.610303, 423.489697) -> (261.610303, 411.610303)
  line L7 (273.489697, 423.489697) -> (261.610303, 423.489697)
  line L8 (0, 444) -> (0, 0)
  line L9 (0, 0) -> (294, 0)
  line L10 (294, 0) -> (294, 444)
  line L11 (294, 444) -> (0, 444)
  circle A1 centre (95.633, 72.5) radius 1.35
  circle A2 centre (144.632832, 130.5) radius 1.35
  circle A3 centre (144.632832, 72.5) radius 1.35
  circle A4 centre (95.633, 130.5) radius 1.35
  line L12 (20.510303, 411.610303) -> (32.389697, 411.610303)
  line L13 (20.510303, 423.489697) -> (20.510303, 411.610303)
  line L14 (32.389697, 423.489697) -> (20.510303, 423.489697)
  line L15 (32.389697, 411.610303) -> (32.389697, 423.489697)
  line L16 (273.489697, 20.510303) -> (273.489697, 32.389697)
  line L17 (261.610303, 20.510303) -> (273.489697, 20.510303)
  line L18 (261.610303, 32.389697) -> (261.610303, 20.510303)
  line L19 (273.489697, 32.389697) -> (261.610303, 32.389697)
  line L20 (200, 319) -> (147, 319)
  line L21 (200, 222) -> (200, 319)
  line L22 (147, 222) -> (200, 222)
  line L23 (147, 319) -> (147, 222)
sketch "Sketch36" plane through (-147, 3, 222) normal (0, 1, 0) x (1, 0, 0)
  line L0 (91.484839, 260.36247) -> (96.484839, 260.36247)
  line L1 (96.484839, 260.36247) -> (96.484839, 230.36247)
  line L2 (96.484839, 230.36247) -> (91.484839, 230.36247)
  line L3 (91.484839, 230.36247) -> (91.484839, 260.36247)
  line L4 (25.162948, 260.36247) -> (30.162948, 260.36247)
  line L5 (30.162948, 260.36247) -> (30.162948, 230.36247)
  line L6 (30.162948, 230.36247) -> (25.162948, 230.36247)
  line L7 (25.162948, 230.36247) -> (25.162948, 260.36247)
  dimension "d161" = 5
  dimension "d162" = 30
  dimension "d163" = 5
  dimension "d164" = 30
  constraints: 16 end point, 4 parallel, 3 coincident, 2 horizontal, 2 perpendicular
  measures "d161" distance of L1.end L2.end
  measures "d162" distance of L0.end L1.end
  measures "d163" distance of L5.end L6.end
  measures "d164" distance of L4.end L5.end
extrude "Extrusion28" cut sketch "Sketch36" against normal through all
body "Solid1"
